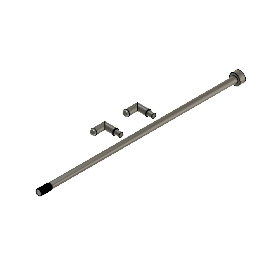
Final N95 UV Storage Container - Accessories v4 (Autodesk Fusion 360 design; units mm, degrees)
Autodesk Fusion 360 part; units mm, degrees
sketch "Sketch1" plane through (0, 0, 0) normal (0, 0, 1) x (1, 0, 0)
  line L0 (0, 0) -> (-10, 0)
  line L1 (-10, 0) -> (-10, -10)
  line L2 (0, 0) -> (5, 0)
  dimension "d1" = 10
  dimension "d2" = 10
  dimension "d7" = 5
  constraint horizontal L0
  constraint coincident L0.start L2.start
  constraint perpendicular L0 L1
  constraint parallel L0 L2
  measures "d1" distance of L0.start L0.end
  measures "d2" distance of L0.end L1.end
  measures "d7" distance of L0.start L2.end
pipe "Pipe1" add diameter 5.5 path "Sketch1" along L0 L1 makes body 1
pipe "Pipe2" add diameter 4 path "Sketch1" along L2 bodies 1
sphere "SpherePrimitive1" add diameter 5.5 placed x (1, 0, 0) y (0, 0, 1) z (0, -1, 0) at (-10, -10, 0) bodies 1
sketch "Sketch3" plane through (0, 0, 0) normal (0, 0, 1) x (1, 0, 0)
  line L0 (35.0025, 0) -> (35.0025, 85)
  line L1 (35.0025, 0) -> (35.0025, -85)
  line L2 (35.0025, 85) -> (35.0025, 90)
  line L3 (35.0025, -85) -> (35.0025, -95)
  line L4 (35.0025, 85) -> (42.5104, 85)
  line L5 (42.5104, 85) -> (29.0024, 85)
  line L6 (35.0025, -85) -> (27.3167, -85)
  line L7 (27.3167, -85) -> (44.8504, -85)
  dimension "d13" = 85
  dimension "d14" = 85
  dimension "d22" = 5
  dimension "d23" = 10
  constraint vertical L0
  constraint parallel L0 L1
  constraint parallel L0 L2
  constraint parallel L1 L3
  constraint perpendicular L2 L4
  constraint perpendicular L2 L5
  constraint perpendicular L3 L6
  constraint perpendicular L3 L7
  measures "d13" distance of L0.start L0.end
  measures "d14" distance of L0.start L1.end
  measures "d22" distance of L0.end L2.end
  measures "d23" distance of L1.end L3.end
pipe "Pipe3" add diameter 5.5 path "Sketch3" along L0 L1 separate body makes body 2
pipe "Pipe4" add diameter 10 path "Sketch3" along L2 bodies 2
pipe "Pipe5" add diameter 5.5 path "Sketch3" along L3 bodies 2
thread "Thread1" "ISO Metric profile 5.5 M5.5x0.5 6g" major diameter 5.427 minor diameter 4.848 pitch 0.5 angle 60 modelled right hand crest width 0.0671 on face at (34.7286, -31.6667, -2.7363) from (35.0025, -85, 0) to (35.0025, -95, 0) crest through (37.716, 85.125, 0) on bodies 2
copy_body "CopyPasteBodies1" bodies 1 makes body 3
move_body "Move1" bodies 3 to x (1, 0, 0) y (0, 1, 0) z (0, 0, 1) at (0, -30, 0)
move_body "Move2" bodies 3 1 to x (1, 0, 0) y (0, 1, 0) z (0, 0, 1) at (21.9751, 18.7571, 0)
copy_body "Body->Comp1" bodies 1 removing the originals makes body 4 in component "Component"
copy_body "Body->Comp2" bodies 3 removing the originals makes body 5 in component "Component'"
copy_body "Body->Comp3" bodies 2 removing the originals makes body 6 in component "Component''"
component "Component" placed x (1, 0, 0) y (0, 1, 0) z (0, 0, 1) at (0, 0, 0)
component "Component'" placed x (1, 0, 0) y (0, 1, 0) z (0, 0, 1) at (0, 0, 0)
component "Component''" placed x (1, 0, 0) y (0, 1, 0) z (0, 0, 1) at (0, 0, 0)
